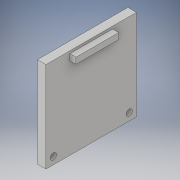
# Autodesk Inventor part: SIM808 Module GSM GPRS GPS Breakout Board SIM808 for Arduino Raspberry
Saved by Autodesk Inventor 2018 (Build 220112000, 112)
## iProperties
Created: 2018-01-27
Part Number: SIM808 Module GSM GPRS GPS Breakout Board SIM808 for Arduino Raspberry
Material: Všeobecné
Document SubType Name: Modeling
Designer: Kuba
Density: 1 g/cm^3
Appearance: Výchozí
Author: Kuba
Autodesk Inventor part; units mm, degrees
ref_plane "YZ Plane" through (0, 0, 0) normal (1, 0, 0) x (0, 1, 0)
ref_plane "XZ Plane" through (0, 0, 0) normal (0, 1, 0) x (-1, 0, 0)
ref_plane "XY Plane" through (0, 0, 0) normal (0, 0, 1) x (1, 0, 0)
sketch "Náčrt1" plane through (0, 0, 0) normal (1, 0, 0) x (0, 1, 0)
  line L0 (0, 0) -> (37, 0)
  line L1 (37, 0) -> (37, -37)
  line L2 (37, -37) -> (0, -37)
  line L3 (0, -37) -> (0, 0)
  circle A0 centre (34, -34) radius 1.25
  circle A1 centre (3, -34) radius 1.25
  dimension "d0" = 37
  dimension "d1" = 37
  dimension "d2" = 2.5
  dimension "d3" = 3
  dimension "d4" = 3
  dimension "d5" = 3
  constraints: 8 end point, 2 centre point, 2 parallel, 1 horizontal, 1 perpendicular
  measures "d0" distance of L2.end L0.start
  measures "d1" distance of L0.start L0.end
  measures "d2" diameter of A0
  measures "d3" distance from line of L1 A0.centre
  measures "d4" distance from line of L2 A0.centre
  measures "d5" distance from line of L3 A1.centre
extrude "Vysunutí1" add sketch "Náčrt1" along normal blind 3.5
sketch "Náčrt2" plane through (3.5, 0, 0) normal (1, 0, 0) x (0, 0, -1)
  line L0 (1, 27.25) -> (3.5, 27.25)
  line L1 (3.5, 27.25) -> (3.5, 9.75)
  line L2 (3.5, 9.75) -> (1, 9.75)
  line L3 (1, 9.75) -> (1, 27.25)
  line L4 (0, 37) -> (37, 37) projected
  line L5 (0, 37) -> (0, 0) projected
  dimension "d8" = 2.5
  dimension "d9" = 17.5
  dimension "d10" = 9.75
  dimension "d11" = 1
  constraints: 8 end point, 2 parallel, 1 horizontal, 1 perpendicular
  measures "d8" distance of L1.end L2.end
  measures "d9" distance of L2.end L0.start
  measures "d10" distance from line of L0.end L4
  measures "d11" distance between parallel lines of L3 L5
extrude "Vysunutí2" add sketch "Náčrt2" along normal blind 2.5
equation "\"d1\" = d0"
equation "\"d4\" = d3"
equation "\"d5\" = d4"
equation "\"d10\" = -0.5 * d9 + 0.5 * d0"
